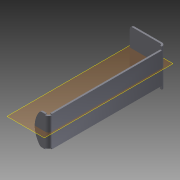
# Autodesk Inventor part: Soporte_Spool_002
Saved by Autodesk Inventor 2015 (Build 190159000, 159)
## iProperties
Created: 2013-09-02
Part Number: Soporte_Spool_002
Material: Stainless Steel
Document SubType Name: Chapa
Designer: Estacion4
Mass: 47.5601 g
Surface Area: 83.595 cm^2
Volume: 5.88615 cm^3
Density: 8.08 g/cm^3
Sheet Metal Rule: Por defecto
Appearance: Steel
Author: Estacion4
Autodesk Inventor part; units mm, degrees
ref_plane "YZ Plane" through (0, 0, 0) normal (1, 0, 0) x (0, 1, 0)
ref_plane "XZ Plane" through (0, 0, 0) normal (0, 1, 0) x (-1, 0, 0)
sketch "Boceto1" plane through (0, 0, 0) normal (0, 0, 1) x (1, 0, 0)
  line L0 (0, -100.2) -> (0, 0)
  line L1 (0, 0) -> (-28.5, 0)
  line L2 (-28.5, 0) -> (-28.5, 1.5)
  line L3 (-28.5, 1.5) -> (1.5, 1.5)
  line L4 (1.5, 1.5) -> (1.5, -101.7)
  line L5 (0, -100.2) -> (-13.5, -100.2)
  line L6 (-13.5, -100.2) -> (-13.5, -101.7)
  line L7 (-13.5, -101.7) -> (1.5, -101.7)
  dimension "d1" = 1.5
  dimension "d2" = 30
  dimension "d8" = 1.5
  dimension "d9" = 1.5
  dimension "d10" = 15
  dimension "d11" = 100.2
  constraints: 16 end point, 4 parallel, 3 perpendicular, 1 coincident, 1 vertical
  measures "d1" distance of L1.end L2.end
  measures "d2" distance of L2.end L3.end
  measures "d8" distance between parallel lines of L4 L0
  measures "d9" distance of L5.end L6.end
  measures "d10" distance of L6.end L4.end
  measures "d11" distance of L0.start L0.end
extrude "Extrusión1" add sketch "Boceto1" along normal mid plane 33
fillet "Empalme1" radius 1.5 2 edges at (0, 0, 0) (0, -100.2, 0)
fillet "Empalme1" radius 3 2 edges at (1.5, 1.5, 0) (1.5, -101.7, 0)
sketch "Boceto2" plane through (-13.5, -101.7, -16.5) normal (0, -1, 0) x (1, 0, 0)
  line L0 (0, 0) -> (12, 0) construction
  arc A0 (7.7463, 30) -> (7.7463, 3) centre (23.832, 16.5) ccw
  line L1 (7.7463, 3) -> (20.0251, 3)
  line L2 (20.0251, 3) -> (20.0251, 0)
  line L3 (20.0251, 33) -> (20.0251, 30)
  line L4 (20.0251, 30) -> (7.7463, 30)
  line L5 (12, 33) -> (12, 0) construction
  line L6 (20.0251, 0) -> (0, 0)
  line L7 (0, 33) -> (20.0251, 33)
  line L8 (12, 33) -> (0, 33) projected
  line L9 (20.0251, 3) -> (20.0251, 5.5)
  line L10 (20.0251, 5.5) -> (5.9434, 5.5)
  line L11 (20.0251, 30) -> (20.0251, 27.5)
  line L12 (20.0251, 27.5) -> (5.9434, 27.5)
  arc A1 (19.332, 34.4444) -> (19.332, -1.4444) centre (23.832, 16.5) ccw construction
  line L13 (0, 33) -> (0, 0)
  point P0 (2.832, 16.5)
  dimension "d14" = 27
  dimension "d23" = 2.5
  dimension "d29" = 2.5
  constraints: 22 end point, 7 perpendicular, 5 point on circle, 3 equal length, 1 centre point, 1 coincident, 1 parallel, 1 vertical, 1 vertical alignment
  measures "d14" distance between parallel lines of L1 L4
  measures "d23" distance of L1.end L9.end
  measures "d29" radial gap between concentric circles of A1 A0
extrude "Extrusión2" cut sketch "Boceto2" against normal blind 100 contours A0 L1 L2 L6 L13 L7 L3 L4
sketch "Boceto4" plane through (-1.5, -101.7, -13.5) normal (0, 0, -1) x (-1, 0, 0)
  arc A0 (-3, 3) -> (0, 0) centre (0, 3) ccw projected
  line L0 (0, 1.5) -> (4.2537, 1.5) projected
  arc A1 (-1.5, 3) -> (0, 1.5) centre (0, 3) ccw projected
  line L1 (0, 0) -> (0, 1.5)
  line L2 (-1.5, 3) -> (-3, 3)
  constraints: 4 end point, 2 perpendicular
extrude "Extrusión4" cut sketch "Boceto4" against normal blind 1
mirror "Simetría2" about plane through (0, 0, 0) normal (0, 0, 1) of "Extrusión4"
fillet "Empalme4" radius 2.5 4 edges at (-5.7537, -100.95, -13.5) (-5.7537, -100.95, 13.5) (-28.5, 0.75, -16.5) (-28.5, 0.75, 16.5)
sketch "Boceto7" plane through (-28.5, 0, -16.5) normal (0, -1, 0) x (1, 0, 0)
  line L0 (0, 33) -> (0, 0) projected
  line L1 (0, 9) -> (15.5, 9)
  line L2 (15.5, 9) -> (15.5, 24)
  line L3 (15.5, 24) -> (0, 24)
  line L4 (0, 24) -> (0, 9)
  line L5 (30, 33) -> (30, 0) projected
  point P0 (0, 16.5)
  point P1 (30, 30)
  point P2 (30, 3)
  dimension "d35" = 15
  dimension "d36" = 14.5
  constraints: 8 end point, 2 midpoint, 2 parallel, 1 horizontal, 1 perpendicular, 1 point on line
  measures "d35" distance between parallel lines of L3 L1
  measures "d36" distance between parallel lines of L2 L5
sketch "Boceto8" plane through (0, 0, 0) normal (0, 0, 1) x (1, 0, 0)
  line L0 (-13, 0) -> (-13, 1.5) projected
  arc A0 (-13, 0) -> (-14.5, -1.5) centre (-13, -1.5) ccw
  line L1 (-14.5, -1.5) -> (-14.5, -6.5)
  line L2 (-14.5, -6.5) -> (-16, -6.5)
  line L3 (-16, -6.5) -> (-16, -1.5)
  arc A1 (-13, 1.5) -> (-16, -1.5) centre (-13, -1.5) ccw
  line L4 (-13, 1.5) -> (-28.5, 1.5) projected
  dimension "d39" = 1.5
  dimension "d40" = 1.5
  dimension "d46" = 8
  constraints: 6 end point, 4 point on circle, 3 tangent, 2 centre point, 2 parallel, 1 perpendicular, 1 point on line
  measures "d39" distance of L1.end L2.end
  measures "d40" radius of A0
  measures "d46" distance between parallel lines of L4 L2
sketch "Boceto6" plane through (-1.5, 1.5, 16.5) normal (0, 1, 0) x (1, 0, 0)
  line L0 (-27, 2.5) -> (-27, 30.5) projected
  circle A0 centre (-22, 16.5) radius 2.5
  point P0 (-26, 2.5)
  point P1 (-26, 30.5)
  point P2 (-27, 16.5)
  dimension "d31" = 5
  dimension "d32" = 5
  constraints: 1 centre point, 1 horizontal alignment, 2 other
  measures "d31" diameter of A0
equation "\"d8\" = d1"
equation "\"d9\" = d8"
equation "\"Radio_pliegue\" = Grosor"
equation "\"Anchura_desahogo_plegado\" = Grosor"
equation "\"Profundidad_desahogo_plegado\" = 0.5 * Grosor"
equation "\"Tamaño_destalonado\" = 4 * Grosor"
equation "\"Remanente_mínimo\" = 2 * Grosor"
equation "\"Radiodetransición\" = Radio_pliegue"
equation "\"Tamaño_de_radio_de_Jacobi\" = Grosor"
equation "\"GapSize\" = Grosor"
equation "\"Grosor\" = 1.5"
body "Solid1"
